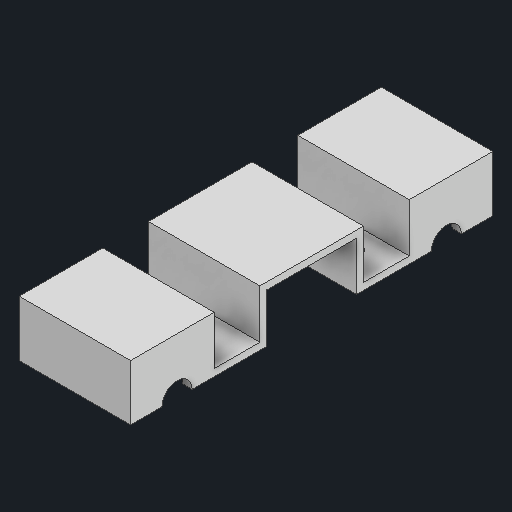
# Autodesk Inventor part: carriage_slider_top
Saved by Autodesk Inventor 2025 (Build 290162010, 162A)
## iProperties
Created: 2024-06-23
Part Number: carriage_slider_top
Material: Generic
Document SubType Name: Modeling
Designer: mihir
Density: 1 g/cm^3
Appearance: Default
Author: mihir
Autodesk Inventor part; units mm, degrees
ref_plane "YZ Plane" through (0, 0, 0) normal (1, 0, 0) x (0, 1, 0)
ref_plane "XZ Plane" through (0, 0, 0) normal (0, 1, 0) x (-1, 0, 0)
sketch "Sketch1" plane through (0, 0, 0) normal (0, 1, 0) x (-1, 0, 0)
  line L0 (0, 0) -> (24, 0)
  line L1 (24, 0) -> (24, -78)
  line L2 (24, -78) -> (0, -78)
  line L3 (0, -78) -> (0, 0)
  dimension "d0" = 78
  dimension "d1" = 24
  constraints: 8 end point, 2 parallel, 1 horizontal, 1 perpendicular
  measures "d0" distance of L2.end L0.start
  measures "d1" distance of L0.start L0.end
extrude "Extrusion1" add sketch "Sketch1" along normal blind 1.5
sketch "Sketch2" plane through (-24, 0, 0) normal (0, 0, 1) x (1, 0, 0)
  line L0 (24, 0) -> (0, 0) projected
  line L1 (0, 0) -> (24, 0)
  line L2 (24, 0) -> (24, 12)
  line L3 (24, 12) -> (0, 12)
  line L4 (0, 12) -> (0, 0)
  line L5 (24, 0) -> (24, 1.5) projected
  dimension "d4" = 12
  constraints: 8 end point, 2 parallel, 1 collinear, 1 horizontal, 1 perpendicular
  measures "d4" distance of L3.end L0.end
extrude "Extrusion2" add sketch "Sketch2" against normal blind 18
sketch "Sketch3" plane through (0, 0, 0) normal (0, -1, 0) x (1, 0, 0)
  line L0 (-2, -10) -> (-22, -10)
  line L1 (-22, -10) -> (-22, -16)
  line L2 (-22, -16) -> (-2, -16)
  line L3 (-2, -16) -> (-2, -10)
  line L4 (-24, 0) -> (0, 0) projected
  line L5 (-24, -78) -> (-24, 0) projected
  line L6 (-2, -13) -> (-22, -13) construction
  line L7 (-12, 0) -> (-12, -78) construction
  line L8 (0, -78) -> (-24, -78) construction
  point P0 (-12, -13)
  dimension "d7" = 20
  dimension "d8" = 6
  dimension "d9" = 16
  constraints: 12 end point, 5 midpoint, 2 parallel, 1 horizontal, 1 perpendicular, 1 point on line
  measures "d7" distance of L0.start L0.end
  measures "d8" distance of L2.end L0.start
  measures "d9" distance between parallel lines of L4 L2
revolve "Revolution1" cut sketch "Sketch3" angle 360 about axis through (-2, 0, -10) along (-1, 0, 0)
ref_plane "Work Plane1" through (-24, 0, -39) normal (0, 0, 1) x (1, 0, 0)
sketch "Sketch4" plane through (0, 0, 0) normal (0, -1, 0) x (1, 0, 0)
  line L0 (0, 0) -> (0, -78) construction
  line L1 (0, -39) -> (-24, -39) construction
  line L2 (-24, -78) -> (-24, -18) construction
  line L3 (-24, -48.65) -> (0, -48.65)
  line L4 (0, -48.65) -> (0, -29.35)
  line L5 (0, -29.35) -> (-24, -29.35)
  line L6 (-24, -29.35) -> (-24, -48.65)
  line L7 (-24, -48.65) -> (0, -29.35) construction
  line L8 (0, -48.65) -> (-24, -29.35) construction
  point P0 (-12, -39)
  dimension "d12" = 19.3
  constraints: 14 end point, 4 midpoint, 3 parallel, 1 collinear, 1 horizontal, 1 perpendicular, 1 point on line
  measures "d12" distance between parallel lines of L3 L5
extrude "Extrusion3" cut sketch "Sketch4" against normal up to surface (1.5 mm away)
sketch "Sketch5" plane through (0, 0, 0) normal (1, 0, 0) x (0, 0, -1)
  line L0 (29.35, 0) -> (29.35, 1.5) projected
  line L1 (29.35, 0) -> (27.85, 0)
  line L2 (27.85, 0) -> (27.85, 10.5)
  line L3 (27.85, 10.5) -> (29.35, 10.5)
  line L4 (29.35, 10.5) -> (29.35, 0)
  line L5 (27.85, 10.5) -> (39, 10.5)
  line L6 (39, 10.5) -> (39, 12)
  line L7 (39, 12) -> (27.85, 12)
  line L8 (27.85, 12) -> (27.85, 10.5)
  point P0 (0, 0)
  point P1 (29.35, 10.5)
  dimension "d15" = 1.5
  dimension "d16" = 10.5
  dimension "d17" = 1.5
  dimension "d18" = 11.15
  constraints: 16 end point, 4 parallel, 2 horizontal, 2 perpendicular
  measures "d15" distance of L2.end L3.end
  measures "d16" distance of L3.end L0.start
  measures "d17" distance of L5.end L6.end
  measures "d18" distance of L6.end L7.end
extrude "Extrusion4" add sketch "Sketch5" against normal up to surface (24 mm away)
sketch "Sketch6" plane through (0, 0, 0) normal (0, -1, 0) x (1, 0, 0)
  line L0 (-2, -16) -> (-22, -16) construction
  line L1 (-24, -29.35) -> (0, -29.35) construction
  line L2 (-2, -16) -> (-22, -16) construction
  line L3 (-22, -16) -> (-22, -29.35) construction
  line L4 (-22, -29.35) -> (-2, -29.35) construction
  line L5 (-2, -29.35) -> (-2, -16) construction
  line L6 (-22, -16) -> (-22, -4) construction
  line L7 (-2, -22.675) -> (-22, -22.675) construction
  line L8 (-17, -22.675) -> (-7, -22.675) construction
  point P0 (0, 0)
  point P1 (-12, -22.675)
  dimension "d21" = 10
  constraints: 12 end point, 4 midpoint, 2 horizontal, 2 parallel, 1 collinear, 1 perpendicular, 1 point on line
  measures "d21" distance of L8.start L8.end
hole "Hole1" at (-7, 0, -22.675) at (-17, 0, -22.675) direction (0, 1, 0) diameter 3 depth 1.5
mirror "Mirror1" about plane through (-24, 0, -39) normal (0, 0, 1) of "Extrusion2", "Revolution1", "Extrusion4", "Hole1"
sketch "Sketch7" plane through (0, 0, 0) normal (1, 0, 0) x (0, 0, -1)
  line L0 (16, 0) -> (4, 0) projected
  arc A0 (13.25, 0) -> (6.75, 0) centre (10, 0) ccw
  line L1 (48.65, 0) -> (78, 0) projected
  arc A1 (71.25, 0) -> (64.75, 0) centre (68, 0) ccw
  arc A2 (16, 0) -> (4, 0) centre (10, 0) ccw projected
  arc A3 (74, 0) -> (62, 0) centre (68, 0) ccw projected
  line L2 (6.75, 0) -> (13.25, 0)
  line L3 (64.75, 0) -> (71.25, 0)
  point P0 (0, 0)
  dimension "d29" = 3.25
  constraints: 4 end point, 4 point on circle, 4 point on line, 2 centre point, 2 concentric, 1 collinear, 1 equal radius, 1 horizontal
  measures "d29" radius of A0
extrude "Extrusion5" cut sketch "Sketch7" against normal up to surface (24 mm away) contours L0 A0 | A1 L1
equation "\"d1\" = slider_top_width"
equation "\"d2\" = slider_top_thickness"
equation "\"d4\" = slider_top_height"
equation "\"d5\" = 2 * bearing_dist - bearing_diameter"
equation "\"d7\" = bearing_length"
equation "\"d8\" = 0.5 * bearing_diameter"
equation "\"d13\" = 2 * bearing_dist - bearing_diameter"
equation "\"d21\" = screw_dist"
equation "\"d22\" = screw_diameter"
equation "\"d29\" = 0.5 * rod_free_tolerance + 0.5 * slider_rod_diameter"
equation "\"slider_top_width\" = 24"
equation "\"slider_top_height\" = 12"
equation "\"slider_top_thickness\" = 1.5"
equation "\"bearing_length\" = 20"
equation "\"bearing_diameter\" = 12"
equation "\"bearing_dist\" = 15"
equation "\"lead_screw_outer_diameter\" = 12"
equation "\"screw_dist\" = 10"
equation "\"screw_diameter\" = 3"
equation "\"slider_rod_diameter\" = 6"
equation "\"rod_free_tolerance\" = 0.5"
body "Solid1"
